Autodesk Fusion 360 part; units mm, degrees
(part 6 of 11)
extrude "Extrude4" cut sketch "Sketch2" against normal blind 3 contours L0 L603 L618 L619 L624 L628 L643 A50 L685 L691 L692 L696 L698 L700 L701 L702 L705 L707 L714 L715 L716 A52 L728 L732 L739 L740 L745 L748 L751 L756 L761 A55 L767 L768 L771 L774 L777 L784 L788 L797 L804 L808 L814 L817 L818 L825 L829 L831 A59 L832 L837 L838 L839 L844 L847 L854 L857 L858 L869 L873 L876 A60 L892 L900 L901 L905 L906 L907 L914 L918 L933 L937 L975 L977 L985 L986 L990 L1001 L1013 L1022 L1024 L1038 L1039 L1041 L1047 L1051 L1054 L1059 A65 L1077 L1080 L1082 L1085 L1091 L1098 L1101 L1102 L1115 A70 L1123 L1132 L1134 L1135 L1137 L1138 L1143 L1174 L1182 L1199 L1212 L1213 L1222 L1223 L1224 L1227 L1232 L1233 L1239 L1247 L1252 L1265 L1268 L1269 L1278 L1283 L1289 L1302 L1306 L1311 L1312 L1313 L1315 A78 L1324 L1327 L1329 A80 L1338 A81 L1341 L1344 L1347 L1348 A85 L1355 L1357 L1360 L1368 L1371 L1376 L1378 L1382 L1389 L1391 L1392 L1393 L1397 L1401 L1402 L1405 L1407 L1408 L1409 A89 L1418 L1419 L1420 L1422 L1426 L1427 L1430 L1431 L1433 L1436 L1438 L1441 L1442 L1444 L1445 L1446 L1447 L1460 L1470 L1471 L1478 L1484 L1485 L1486 L1498 L1499 L1501 L1502 L1507 L1511 L1541 L1548 L1552 L1556 L1572 L1574 L1575 L1582 L1585 L1586 L1587 L1588 L1596 A100 L1598 L1599 L1608 L1612 L1613 L1615 L1617 L1620 L1621 L1624 L1625 A102 L1632 L1634 L1635 L1637 L1638 L1641 L1642 L1644 L1645 L1647 L1650 L1652 L1655 L1659 L1660 L1662 L1664 L1666 L1669 L1671 L1672 L1673 L1674 L1676 L1677 L1678 L1681 L1682 L1687 L1688 A107 L1697 A108 L1699 L1700 L1710 L1711 L1713 L1714 L1715 L1716 L1718 L1719 L1722 L1723 L1726 L1728 L1729 L1730 L1731 L1735 L1736 A109 L1739 L1740 L1741 L1742 L1745 L1746 L1747 L1748 L1749 L1751 L1752 L1753 L1757 L1758 L1759 L1761 L1764 L1765 L1767 L1769 L1773 L1775 L1777 L1780 L1786 L1788 L1789 L1790 L1791 L1792 L1794 L1795 A114 L1797 A115 L1799 L1800 A116 A117 L1804 L1807 L1813 L1814 L1818 L1819 L1820 L1821 L1822 L1823 L1824 L1825 L1826 A119 L1827 L1828 L1829 L1830 L1831 L1832 L1833 A120 L1834 L1835 L1836 L1837 L1838 L1839 L1840 L1841 L1842 L1843 L1844 L1845 L1846 L1847 L1848 A121 L1849 L1850 L1851 L1852 L1853 L1854 L1855 L1856 A122 L1857 L1858 L1859 L1860 L1861 L1862 L1863 L1864 L1865 A123 L1866 L1867 L1868 L1869 L1870 L1871 L1872 L1873 L1874 L1875 L1876 A124 L1879 L1881 L1882 L1883 L1886 L1894 L1895 A126 L1904 L1905 L1906 L1910 L1918 L1919 L1921 L1922 L1923 L1925 L1932 L1934 L1935 L1936 L1937 L1938 L1939 A128 L1940 L1941 L1942 L1943 L1944 L1945 L1946 L1947 L1948 L1949 L1950 L1951 L1952 L1953 L1954 L1955 L1956 L1957 L1958 L1959 L1960 L1961 L1962 L1963 L1964 L1966 L1967 L1968 L1969 L1970 L1971 L1972 L1973 A129 L1974 L1975 L1976 L1977 L1978 L1979 L1980 L1981 L1982 L1983 L1984 L1985 L1986 L1987 A130 L1988 L1989 L1990 L1991 L1992 L1993 L1994 L1995 L1997 L1998 L2002 L2003 A131 L2004 L2006 L2007 L2009 L2011 L2012 L2013 L2014 L2016 L2017 L2021 L2023 L2024 L2025 L2026 L2027 L2028 L2030 L2031 L2032 L2033 L2034 L2035 L2036 L2037 L2038 L2039 L2040 L2041 L2042 L2045 A132 L2047 L2048 L2049 L2050 L2051 L2053 A133 L2055 L2056 L2057 L2060 L2062 L2063 L2064 L2066 L2067 L2069 L2071 L2072 L2073 L2074 L2075 L2076 L2077 L2078 L2080 L2081 L2082 L2084 L2085 L2086 L2088 L2089 L2091 L2092 L2095 L2096 L2097 L2098 L2099 L2100 L2103 L2104 L2105 L2106 L2107 L2111 L2113 L2114 L2115 L2116 L2117 L2118 L2119 L2120 L2121 L2122 L2123 L2124 L2125 L2126 L2129 L2130 L2131 L2133 L2134 L2135 L2136 A134 L2137 L2138 L2139 L2140 L2141 L2142 L2143 L2144 L2147 L2148 L2149 L2151 L2152 L2153 A135 L2155 L2156 L2157 A136 L2159 L2160 L2161 L2162 L2163 L2164 L2165 L2166 A137 L2167 L2169 L2171 L2172 L2173 L2174 L2175 L2176 L2178 L2179 L2180 L2181 L2182 L2184 L2185 L2186 L2188 L2189 L2190 L2191 L2192 L2193 L2194 L2195 L2196 L2197 L2198 A138 L2199 L2200 L2201 L2202 A140 A141 L2205 L2206 L2207 L2208 L2209 L2210 L2211 L2212 L2213 L2214 L2215 L2216 L2217 L2218 L2220 L2221 L2223 L2224 L2225 L2226 L2227 L2228 L2229 A142 L2230 L2233 L2234 L2235 L2236 L2237 L2238 A144 L2239 L2240 L2241 L2242 L2243 L2244 L2245 L2246 L2247 L2248 L2249 L2250 L2251 L2252 L2253 L2254 L2255 L2256 L2257 A145 L2258 L2259 L2260 L2261 L2262 L2263 L2264 L2265 L2266 L2267 L2268 L2269 L2270 L2271 L2272 L2273 L2274 L2275 A147 L2276 L2277 L2278 L2279 L2280 L2281 L2282 L2283 L2284 L2285 L2286 L2287 L2288 L2289 L2290 L2291 L2292 L2293 A149 L2294 L2295 L2296 A150 L2297 L2298 L2299 L2300 L2301 L2302 L2303 L2304 L2305 L2306 L2307 A151 L2308 L2309 L2310 L2311 L2312 L2313 L2314 L2315 L2316 L2317 L2318 L2319 L2320 L2321 L2322 L2323 L2324 L2325 L2326 L2327 L2328 L2329 L2330 L2331 L2332 L2333 L2334 L2335 L2336 L2337 L2338 L2883 L2884 L2885 L2886 L2887 L2888 L2889 L2890 L2891 A183 A200 L3160 L3161 L3162 L3163 L3164 L3165 L3166 L3167 L3168 | L0 L3 L619 L628 L643 L685 L1022 L1024 A65 L1077 L1080 L1082 L1085 L1091 L1098 L1101 L1102 L1115 A70 L1123 L1132 L1134 L1135 L1137 L1138 L1143 L1174 L1182 L1199 L1212 L1213 L1222 L1223 L1224 L1227 L1232 L1233 L1239 L1247 L1252 L1265 L1268 L1269 L1278 L1283 L1289 L1302 L1306 L1311 L1312 L1313 L1315 A78 L1324 L1327 L1329 L1338 A81 L1341 L1344 L1347 L1348 L1355 L1357 L1360 L1368 L1371 L1376 L1378 L1382 L1391 L1392 L1393 L1397 L1401 L1402 L1405 L1407 L1408 L1409 A89 L1418 L1420 L1422 L1427 L1430 L1433 L1438 L1441 L1444 L1445 L1446 L1447 L1460 L1470 L1471 L1478 L1484 L1485 L1486 L1498 L1499 L1501 L1502 L1507 L1728 L1731 L1736 L1746 L1747 L1749 L1751 L1758 L1764 L1777 L1789 L1794 L1795 L1799 A116 L1804 L1807 L1813 L1814 L1834 A124 L1882 A126 L1905 L1922 L1939 A128 L1941 L1942 L1944 L1947 L1948 L1949 L1950 L1951 L1952 L1954 L1955 L1956 L1957 L1966 L1967 L1971 L1973 L1974 L1977 L1978 L1980 L1981 L1983 L1984 L1985 L1986 A130 L1988 L1989 L1991 L1992 L1994 L1997 L2026 L2032 L2040 L2062 L2063 L2064 L2080 L2081 L2082 L2086 L2103 L2105 L2106 L2107 L2114 L2115 L2116 L2117 L2119 L2120 L2121 L2122 L2123 L2124 L2125 L2126 L2129 L2130 L2131 L2133 L2134 L2135 L2136 A134 L2137 L2138 L2139 L2140 L2141 L2142 L2143 L2144 L2147 L2148 L2149 L2151 L2152 L2153 A135 L2155 L2156 L2157 A136 L2159 L2160 L2161 L2162 L2163 L2164 L2165 L2166 A137 L2167 L2169 L2171 L2172 L2173 L2174 L2175 L2176 L2178 L2179 L2180 L2181 L2182 L2184 L2185 L2186 L2193 L2194 L2195 L2196 L2197 L2198 A138 L2199 L2200 L2201 L2202 L2205 L2207 L2208 L2209 L2210 L2211 L2212 L2214 L2215 L2216 L2217 L2218 L2220 L2224 L2225 L2230 L2233 L2234 L2235 L2236 L2237 L2238 A144 L2254 L2255 L2256 L2257 A145 L2258 L2262 L2263 L2267 L2268 L2269 L2270 L2271 L2273 L2274 L2275 L2276 L2278 L2279 L2280 L2281 L2282 L2283 L2284 L2285 L2291 L2292 L2293 A149 L2294 L2295 A150 L2297 L2298 L2299 L2300 L2301 L2302 A151 L2308 L2309 L2320 L2321 L2324 L2331 L2332 L2333 L2436 L2437 L2438 A158 A173 L2690 L2691 L2692 L2693 L2694 A174 L2695 L2696 L2697 L2698 L2699 L2700 L2701 L2702 L2703 L2704 A175 L2705 L2706 L2707 L2708 L2709 L2727 L2728 L2729 L2730 L2731 A176 L2732 L2733 L2734 L2735 L2736 L2737 L2738 L2739 L2740 L2741 A177 L2742 L2743 L2744 L2745 L2746 L2764 L2765 L2766 L2767 L2768 A178 L2769 L2770 L2771 L2772 L2773 L2774 L2775 L2776 L2777 L2778 A179 L2779 L2780 L2781 L2782 L2783 L2801 L2802 L2803 L2804 L2805 A180 L2806 L2807 L2808 L2809 L2810 L2811 L2812 L2813 L2814 L2815 A181 L2816 L2817 A200 | L0 L1820 L1821 L1822 L1823 L1824 A119 L1829 L1830 L1833 A120 L1836 L1837 L1838 L1839 L1842 L1843 L1844 L1845 L1848 L1849 L1850 L1852 L1855 L1858 L1859 L1860 L1861 L1862 L1865 A123 L1866 L1867 L1868 L1869 L1873 L1876 L2260 L2261 L2264 L2265 L2266 L2272 A147 L2277 L2286 L2287 L2288 L2289 L2296 L2303 L2304 L2306 L2307 L2310 L2312 L2313 L2314 L2315 L2316 L2317 L2318 L2322 L2323 L2325 L2328 L2329 L2330 L2334 L2335 L2336 L2337 L2338 L2462 L2463 A159 L2464 L2465 L2466 L2467 L2468 L2469 L2470 L2471 L2472 L2473 A160 L2474 L2475 | L0 L603 L618 L624 A50 L691 L692 L696 L698 L700 L701 L702 L705 L707 L714 L715 L716 A52 L728 L732 L739 L740 L745 L748 L751 L756 L761 A55 L767 L768 L771 L774 L777 L784 L788 L797 L804 L808 L814 L817 L818 L825 L829 L831 A59 L832 L837 L838 L839 L844 L847 L854 L857 L858 L869 L873 L876 A60 L892 L900 L901 L905 L906 L907 L914 L918 L933 L937 L975 L977 L985 L986 L990 L1001 L1013 L1038 L1039 L1041 L1047 L1051 L1054 L1059 A80 A85 L1511 L1541 L1572 L1574 L1575 L1582 L1585 L1586 L1587 L1588 A100 L1598 L1608 L1612 L1613 L1615 L1620 L1621 L1624 L1625 A102 L1632 L1634 L1635 L1637 L1638 L1641 L1642 L1644 L1645 L1647 L1650 L1652 L1655 L1659 L1660 L1662 L1664 L1666 L1669 L1671 L1672 L1673 L1674 L1676 L1677 L1678 L1681 L1682 L1687 L1688 A107 L1697 A108 L1699 L1700 L1710 L1711 L1713 L1714 L1715 L1716 L1718 L1719 L1722 L1723 L1726 L1729 L1735 L1739 L1740 L1741 L1742 L1745 L1752 L1753 L1759 L1786 L1792 L1800 L1818 L1819 L1825 L1827 L1828 L1835 L1840 L1846 L1847 A121 L1851 L1853 L1854 L1856 A122 L1857 L1863 L1864 L1870 L1871 L1874 L1879 L1881 L1883 L1886 L1894 L1895 L1904 L1906 L1910 L1918 L1919 L1921 L1923 L1925 L1932 L1934 L1936 L1937 L1938 L1940 L1943 L1945 L1946 L1953 L1958 L1959 L1960 L1962 L1963 L1964 L1968 L1969 L1970 L1972 A129 L1975 L1976 L1979 L1982 L1987 L1990 L1993 L1995 L1998 L2002 A131 L2004 L2006 L2007 L2009 L2011 L2012 L2013 L2014 L2016 L2017 L2021 L2023 L2025 L2028 L2030 L2031 L2033 L2034 L2036 L2037 L2038 L2039 L2041 L2045 A132 L2047 L2048 L2051 A133 L2055 L2056 L2057 L2060 L2066 L2067 L2069 L2071 L2072 L2073 L2074 L2075 L2076 L2077 L2078 L2084 L2085 L2088 L2089 L2091 L2092 L2095 L2096 L2097 L2098 L2099 L2100 L2104 L2111 L2113 L2118 L2188 L2189 L2190 L2191 L2192 A140 A141 L2206 L2213 L2221 L2223 L2226 L2227 L2228 L2229 A142 L2239 L2240 L2241 L2242 L2243 L2244 L2245 L2246 L2247 L2248 L2249 L2250 L2251 L2252 L2253 L2290 A161 L2489 L2490 L2491 L2492 L2493 L2494 L2495 L2496 L2497 L2498 L2499 L2500 L2501 L2502 L2503 A162 L2504 L2505 L2506 L2507 L2508 L2509 L2510 L2511 L2512 L2513 A163 L2514 L2515 L2516 L2517 L2518 L2519 L2520 L2521 L2522 L2523 L2524 L2525 L2526 L2527 L2528 L2529 L2530 L2531 L2532 L2533 L2534 L2535 L2536 L2537 L2538 L2539 L2540 A164 L2541 L2542 L2543 L2544 L2545 L2546 L2547 L2548 L2549 L2550 A165 L2551 L2552 L2553 L2554 L2555 L2556 L2557 L2558 L2559 L2560 L2561 L2562 L2563 L2564 L2565 L2566 L2567 L2568 L2569 L2570 L2571 L2572 L2573 L2574 L2575 L2576 L2577 A166 L2578 L2579 L2580 L2581 L2582 L2583 L2584 L2585 L2586 L2587 A167 L2588 L2589 L2590 L2591 L2592 L2593 L2594 L2595 L2596 L2597 L2598 L2599 L2600 L2601 L2602 L2603 L2604 L2605 L2606 L2607 L2608 L2609 L2610 L2611 L2612 L2613 L2614 A168 L2615 L2616 L2617 L2618 L2619 L2620 L2621 L2622 L2623 L2624 A169 L2625 L2626 L2627 L2628 L2629 L2630 L2631 L2632 L2633 L2634 L2635 L2636 L2637 L2638 L2639 A170 A183 | L3 A2 A3 L223 L238 L240 A19 L245 A20 L246 L337 L338 L341 L343 L344 L345 L346 L347 L348 L350 L352 L385 L386 L387 L388 L389 L390 L391 L392 L393 L394 L395 L396 L397 L398 L399 L400 L403 L405 L407 L413 L414 L415 L416 A32 L417 L418 L419 L420 L421 A33 L422 L423 L424 L425 L428 L429 L430 L432 L433 L434 L435 L441 L442 L443 A34 L445 L446 L447 L450 L451 L452 L453 L454 L455 L456 L457 L459 L460 L462 L463 L464 L466 A35 L467 L468 L469 L470 L471 L472 L473 L474 L475 L476 L477 L478 L479 L480 L481 L482 L497 L498 L499 L500 L501 L502 L503 L504 L505 L506 L507 L508 L509 L510 L511 L512 L513 L514 L515 L516 L625 L638 L639 L763 L764 L769 L775 A56 L798 L811 L815 L816 L820 L821 A58 L824 L826 L828 L830 L833 L835 L845 L849 L852 L859 L861 L862 L863 L866 L867 L870 L875 L883 L891 L893 L898 L908 L911 L915 L919 L921 L929 L934 L1020 L1034 L1044 L1050 L1052 L1058 L1066 L1078 L1079 L1083 L1086 L1087 L1088 L1089 L1092 A67 L1093 L1094 L1095 L1096 L1099 L1103 L1107 L1108 L1110 L1111 L1112 L1113 L1114 L1118 A69 L1122 L1124 L1125 L1126 L1127 L1128 L1129 L1130 L1131 L1136 L1144 L1145 L1147 L1148 L1151 L1152 A71 L1155 L1157 A72 L1168 L1170 L1173 L1177 L1178 L1179 L1181 L1187 L1188 L1195 L1200 L1204 L1206 L1207 L1211 L1214 L1216 L1218 L1221 L1225 L1230 L1236 L1246 L1248 L1253 L1275 L1296 L1888 A125 A127 L1924 A173 A193 L3056 L3057 L3058 L3059 L3060 A194 L3061 L3062 L3063 L3064 L3065 L3066 L3067 L3068 L3069 L3070 A195 L3071 L3072 L3073 L3074 L3075 L3093 L3094 L3095 L3096 L3097 A196 L3098 L3099 L3100 L3101 L3102 L3103 L3104 L3105 L3106 L3107 A197 L3108 L3109 L3110 L3111 L3112 L3130 L3131 L3132 L3133 L3134 A198 L3135 L3136 L3137 L3138 L3139 L3140 L3141 L3142 L3143 L3144 A199 L3145 L3146 L3147 L3148 L3149 A200 A222 | A124 A125 A126 A127 A173 A200 | L2 L77 L80 L81 L84 L85 L89 L123 L124 L125 L126 L127 L128 L129 L130 L131 L132 L133 L134 L135 L136 L137 L138 L139 L140 L141 L142 L143 L144 L145 L146 L147 L148 L149 L150 A8 A10 L185 L187 A12 L188 A13 L190 L191 L192 L193 L194 L195 L196 A14 L197 L198 L199 L200 L201 L202 L203 L204 L205 L206 L207 L208 L209 L210 A15 L211 L212 L213 L214 L215 L216 L217 L218 L219 L220 L221 L224 L225 L226 L227 L228 L229 L230 L231 L232 L233 L234 L235 L236 L249 L250 L251 L252 L253 L254 L255 L256 L257 L258 L259 L260 A36 L544 A39 L545 L571 L572 L620 L621 L631 L633 L637 A46 A47 L641 L656 L663 L671 L674 L693 L695 L703 L706 L709 L711 L713 L724 L726 L727 L730 L733 L738 L741 L746 A53 L749 L750 A54 L754 L755 L757 L758 L759 L760 L762 L766 L770 L772 L773 L776 L778 L779 L780 L781 L782 L786 L787 L789 L791 L792 L793 L794 L795 L796 L799 L800 L801 L802 L803 A57 L805 L806 L807 L809 L810 L812 L813 L819 L822 L823 L827 L834 L836 L840 L841 L843 L846 L848 L850 L851 L853 L855 L860 L864 L865 L868 L871 L872 L874 L877 L879 L899 L902 L909 L913 L917 L920 L930 L931 L944 L945 L1081 L1084 A66 A68 L1097 L1105 L1109 L1116 L1119 L1120 L1121 L1133 L1139 L1140 L1141 L1142 L1146 L1153 L1156 L1160 L1161 L1162 L1163 L1164 L1166 L1167 L1169 L1172 L1176 L1183 L1184 L1185 L1186 L1189 L1190 L1191 L1192 L1193 L1196 L1197 A73 L1201 L1203 L1208 L1209 L1210 L1215 L1217 L1219 L1220 L1226 L1228 L1229 L1234 L1237 L1240 L1241 L1242 L1243 L1244 L1245 L1249 L1251 L1255 L1273 A77 A90 L1440 L1483 L1503 L2376 L2377 L2378 L2379 L2380 L2381 L2384 L2385 L2386 L2387 L2388 A154 L2389 L2390 L2391 L2392 L2393 L2394 L2395 L2396 L2397 L2398 L2399 L2400 L2401 L2403 L2404 L2406 A155 L2407 L2408 L2409 L2410 L2411 L2412 L2413 L2414 L2415 L2417 L2418 L2420 L2421 A190 L3216 L3217 L3218 L3219 L3220 L3221 L3222 L3223 L3224 L3225 L3226 L3227 A202 L3228 L3229 L3230 L3231 L3232 L3233 L3234 L3235 L3236 L3237 A203 L3238 L3239 L3240 L3241 L3242 L3243 L3244 L3245 L3246 L3247 L3248 L3249 L3250 L3251 L3252 L3253 L3254 L3255 L3256 L3257 L3258 L3259 L3260 L3261 L3262 L3263 L3264 A204 L3265 L3266 L3267 L3268 L3269 L3270 L3271 L3272 L3273 L3274 A205 L3275 L3276 L3277 L3278 L3279 L3280 L3281 L3282 L3283 L3284 L3285 L3286 L3287 L3288 L3289 L3290 L3291 L3292 L3293 L3294 L3295 L3296 L3297 L3298 L3299 L3300 L3301 A206 L3302 L3303 L3304 L3305 L3306 L3307 L3308 L3309 L3310 L3311 A207 L3312 L3313 L3314 L3315 L3316 L3317 L3318 L3319 L3320 L3321 L3322 L3323 L3324 L3325 L3326 L3327 L3328 L3329 L3330 L3331 L3332 L3333 L3334 L3335 L3336 L3337 L3338 A208 L3339 L3340 L3341 L3342 L3343 L3344 L3345 L3346 L3347 L3348 A209 L3349 L3350 L3351 L3352 L3353 L3354 L3355 L3356 L3357 L3358 L3359 L3360 L3361 L3362 L3363 A210 A225 L3595 L3596 L3597 | L1387 L1390 L1412 L1423 L1424 L1435 L1437 L1443 L1877 L1880 L1884 L1887 L1891 L1892 A125 L1893 L1896 L1901 L1903 L1911 L1912 L1913 A127 L1916 L1917 L1926 L1929 L1930 L1931 L1933 L2671 L2672 L2673 L2674 L2675 L2676 L2677 L2678 L2679 A173 | A2 A3 L29 L30 L34 L37 L40 L43 L98 L107 L116 L117 L122 L171 A9 A11 L222 L223 L237 L238 L239 L240 L241 L242 L243 A18 A19 L244 L245 A20 L246 A21 L247 L248 L261 L262 L266 L268 L270 L271 L272 L273 L274 L275 L276 L277 L278 L279 L280 L281 L282 L283 L284 L285 L286 L287 L288 L289 L290 L291 L292 L294 A22 L295 L296 A23 L297 L298 L299 L300 L301 L302 L303 L304 L305 L306 L307 L308 L309 L310 L311 L312 L313 L314 L315 L316 A24 L317 L318 A25 L319 L320 L321 L322 L323 A26 L324 L325 L326 L327 L328 L329 L330 A27 L331 L332 L333 L334 L335 L336 L337 L338 L339 A28 L340 L341 L342 L343 L344 L345 L346 L347 L348 L349 L350 L351 L352 L353 L354 L355 L356 L357 L358 L359 L360 L361 L362 L363 L364 L365 L366 L367 L368 L369 L370 L371 L372 L373 L374 L375 L376 L377 L379 L380 L382 L383 L384 L385 L386 L387 L388 L389 L390 L391 L392 L393 L394 L395 L396 L397 L398 L399 L400 L401 L402 L403 L404 L405 L406 L407 L408 L409 L410 L411 L412 A31 L413 L414 L415 L416 A32 L417 L418 L419 L420 L421 A33 L422 L423 L424 L425 L428 L429 L430 L432 L433 L434 L435 L441 L442 L443 A34 L445 L446 L447 L450 L451 L452 L453 L454 L455 L456 L457 L459 L460 L462 L463 L464 L466 A35 L467 L468 L469 L470 L471 L472 L473 L474 L475 L476 L477 L478 L479 L480 L481 L482 L497 L498 L499 L500 L501 L502 L503 L504 L505 L506 L507 L508 L509 L510 L511 L512 L513 L514 L515 L516 L546 L547 L548 L549 L550 L551 L552 L553 L554 L555 L556 L557 L558 L559 L562 L563 L565 A41 L566 A42 L573 L578 L581 L582 L585 L586 L587 L589 L590 L591 L592 L594 L596 L597 L598 L600 L601 L604 L605 L606 L608 L609 L610 L611 L612 L615 L625 L638 L639 L644 L645 L647 L648 L649 L650 L651 A48 L652 L654 L655 L658 L659 L665 L666 L667 L668 L669 L670 L672 L673 L675 L676 L677 L678 L679 L681 L682 L683 L684 L686 A51 L687 L688 L690 L718 L720 L721 L725 L729 L735 L737 L747 L753 L763 L764 L765 L769 L775 L790 A56 L798 L811 L815 L816 L820 L821 A58 L824 L826 L828 L830 L833 L835 L845 L849 L852 L859 L861 L862 L863 L866 L867 L870 L875 L881 L883 L884 L891 L893 L898 L908 L911 L915 L919 L921 L929 L934 L939 L940 L941 L942 L943 L946 L950 L951 L953 A62 L956 L960 L961 L962 L964 L965 L968 L969 L970 L976 L978 L981 L987 A63 L988 L991 L992 L993 L997 L1000 L1002 L1003 L1006 L1007 L1009 L1011 L1012 L1014 L1020 L1034 L1036 L1044 L1050 L1052 L1056 L1058 L1060 L1066 L1068 L1078 L1079 L1083 L1086 L1087 L1088 L1089 L1092 A67 L1093 L1094 L1095 L1096 L1099 L1103 L1107 L1108 L1110 L1111 L1112 L1113 L1114 L1118 A69 L1122 L1124 L1125 L1126 L1127 L1128 L1129 L1130 L1131 L1136 L1144 L1145 L1147 L1148 L1149 L1150 L1151 L1152 A71 L1154 L1155 L1157 L1158 A72 L1159 L1165 L1168 L1170 L1171 L1173 L1175 L1177 L1178 L1179 L1181 L1187 L1188 L1195 L1200 L1204 L1206 L1207 L1211 L1214 L1216 L1218 L1221 L1225 L1230 L1236 L1246 L1248 L1253 L1254 L1261 L1275 L1276 L1296 L1314 L1322 A79 A82 L1340 L1346 A84 A86 L1374 L1403 L1411 L1416 L1434 L1435 L1443 L1527 L1546 L1551 L1570 L1584 L1589 L1602 L1623 A110 A118 L1888 A125 A127 L1924 L2010 L2015 L2029 L2046 L2359 A170 L2640 L2641 L2642 L2643 L2644 L2645 L2646 L2647 L2648 L2671 L2672 L2673 L2674 L2675 L2676 L2677 L2678 L2679 A173 A222 L3555 L3556 L3557 L3558 L3559 L3560 L3561 L3562 L3563 L3586 L3587 L3588 L3589 L3590 L3591 L3592 L3593 L3594 A225 | L1388 L1389 L1398 L1417 L1421 L1428 L1429 L1442 A124 L1889 L1890 L1892 L1896 L1897 L1898 A126 L1899 L1900 L1902 L1903 L1907 L1911 L1915 L1917 L1920 L1927 L1928 L1929 L1931 L1933 A200 L3160 L3161 L3162 L3163 L3164 L3165 L3166 L3167 L3168 | L2 L4 L5 L6 L7 L8 L9 L10 L11 L12 L13 L14 L15 A0 A1 L22 L32 L36 L38 L42 L44 L49 L52 L54 L75 L76 L77 A4 A5 L78 L79 L80 L81 L82 L83 L84 L85 A6 L86 L87 L88 L89 L90 A7 L91 L92 L106 L112 L114 L120 L121 L123 L124 L125 L126 L127 L128 L129 L130 L131 L132 L133 L134 L135 L136 L137 L138 L139 L140 L141 L142 L143 L144 L145 L146 L147 L148 L149 L150 L151 L152 L153 L154 L155 L156 L172 A8 A10 L185 L187 A12 L188 A13 L190 L191 L192 L193 L194 L195 L196 A14 L197 L198 L199 L200 L201 L202 L203 L204 L205 L206 L207 L208 L209 L210 A15 L211 L212 L213 L214 L215 L216 L217 L218 L219 L220 L221 L224 L225 L226 L227 L228 L229 L230 L231 L232 L233 L234 L235 L236 L249 L250 L251 L252 L253 L254 L255 L256 L257 L258 L259 L260 L517 L518 L519 L520 L521 L522 L523 L525 L526 L527 L528 L530 L531 L532 L535 L537 L538 L539 A36 L541 L542 L543 A37 L544 A38 A39 L545 L560 A40 L561 L564 L567 L568 L569 L571 L572 L574 L575 L576 L577 L579 L580 L583 L584 A43 L588 L593 L595 L599 L602 L607 L613 L614 L616 L620 L621 L629 L631 L632 L633 L635 L636 L637 A46 A47 L641 L646 L656 L662 L663 L671 L674 A49 L689 L693 L695 L703 L706 L709 L711 L713 L724 L726 L727 L730 L733 L738 L741 L746 A53 L749 L750 A54 L754 L755 L757 L758 L759 L760 L762 L766 L770 L772 L773 L776 L778 L779 L780 L781 L782 L786 L787 L789 L791 L792 L793 L794 L795 L796 L799 L800 L801 L802 L803 A57 L805 L806 L807 L809 L810 L812 L813 L819 L822 L823 L827 L834 L836 L840 L841 L843 L846 L848 L850 L851 L853 L855 L860 L864 L865 L868 L871 L872 L874 L877 L879 L899 L902 L909 L913 L917 L920 L930 L931 L944 L945 L955 L958 L959 L963 L966 L967 L971 L973 L974 L979 L983 L1004 L1005 L1016 L1017 L1018 L1019 L1028 L1029 L1030 L1032 L1035 L1037 L1045 L1046 L1048 L1049 L1055 L1057 L1062 L1063 L1064 L1065 L1067 L1069 L1071 L1074 L1075 L1076 L1081 L1084 A66 A68 L1097 L1105 L1109 L1116 L1119 L1120 L1121 L1133 L1139 L1140 L1141 L1142 L1146 L1153 L1156 L1160 L1161 L1162 L1163 L1164 L1166 L1167 L1169 L1172 L1176 L1183 L1184 L1185 L1186 L1189 L1190 L1191 L1192 L1193 L1196 L1197 A73 L1198 L1201 L1203 L1208 L1209 L1210 L1215 L1217 L1219 L1220 L1226 L1228 L1229 L1231 L1234 L1235 L1237 L1240 L1241 L1242 L1243 L1244 L1245 L1249 L1251 L1255 L1257 L1264 L1266 L1270 L1271 L1273 L1277 L1280 L1282 L1285 A77 L1291 L1294 L1295 L1297 L1298 L1299 L1300 L1301 L1303 L1304 L1305 L1308 L1309 L1317 L1319 L1323 L1325 L1326 L1328 L1331 L1332 L1333 L1334 L1336 L1337 L1339 L1342 L1343 L1345 L1349 A83 L1350 L1351 L1353 L1359 L1361 L1362 L1363 L1364 L1365 L1366 A88 L1370 L1372 L1373 L1375 L1377 L1379 L1380 L1381 L1383 L1384 L1385 L1386 L1396 L1400 L1404 L1410 L1413 L1414 L1415 L1425 A90 L1439 A91 L1440 L1449 L1450 A92 L1452 L1453 L1455 L1456 L1457 L1461 L1464 L1465 L1466 L1468 L1469 L1473 L1474 L1475 A93 L1479 L1480 L1481 L1482 L1483 L1487 L1488 L1491 L1492 L1493 L1496 A94 L1500 L1503 L1505 L1508 L1509 L1513 L1514 L1515 L1517 A96 L1518 L1519 L1520 L1522 L1523 L1524 A97 A98 L1528 L1531 L1533 L1534 L1536 L1537 L1540 L1545 L1547 L1549 L1550 L1553 L1554 L1555 L1557 L1562 L1563 L1564 L1565 L1567 L1569 L1571 L1573 L1578 L1581 L1583 L1590 L1591 L1592 L1597 L1600 L1603 L1604 L1606 L1607 L1609 L1610 A101 L1618 L1622 L1626 L1627 L1628 L1629 L1630 L1631 L1633 L1636 L1639 L1640 L1643 L1646 A103 L1648 L1649 L1651 L1653 L1654 L1656 L1657 L1658 L1661 L1663 L1665 L1667 L1668 A104 A105 L1670 L1675 L1679 L1680 L1683 L1684 L1685 L1686 L1689 L1690 L1695 L1696 L1698 L1701 L1703 L1705 L1706 L1709 L1717 L1720 L1721 L1724 L1725 L1733 L1734 L1737 L1738 L1743 L1750 L1754 L1755 L1756 L1760 L1762 L1763 A111 L1766 L1768 L1770 L1771 L1772 L1776 L1778 A112 L1779 L1782 L1783 L1784 L1787 L1796 L1798 L1801 L1802 L1803 L1805 L1808 L1809 L1810 L1811 L1812 L1815 L1817 L2339 L2340 L2341 L2342 L2343 A152 L2344 L2345 L2346 L2347 L2348 A153 L2349 L2350 L2351 L2352 L2353 L2354 L2355 L2356 L2357 L2358 L2360 L2361 L2362 L2363 L2364 L2365 L2366 L2367 L2368 L2369 L2370 L2371 L2372 L2373 L2374 L2375 L2376 L2377 L2378 L2379 L2380 L2381 L2382 L2383 L2384 L2385 L2386 L2387 L2388 A154 L2389 L2390 L2391 L2392 L2393 L2394 L2395 L2396 L2397 L2398 L2399 L2400 L2401 L2403 L2404 L2406 A155 L2407 L2408 L2409 L2410 L2411 L2412 L2413 L2414 L2415 L2417 L2418 L2420 L2421 L2422 L2423 L2426 L2429 L2431 L2433 L2434 L2435 A190 L3006 L3007 L3008 L3009 L3010 L3011 L3012 L3013 L3014 L3037 L3038 L3039 L3040 L3041 L3042 L3043 L3044 L3045 A193 | L1387 L1388 L1389 L1390 L1398 L1412 L1417 L1421 L1423 L1424 L1428 L1429 L1435 L1437 L1442 L1443 L1877 L1880 L1884 L1887 L1889 L1890 L1891 L1893 L1897 L1898 L1899 L1900 L1901 L1902 L1907 L1912 L1913 L1915 L1916 L1920 L1926 L1927 L1928 L1930 L2667 L2668 L2669 L2670 L3169 L3170 L3171 L3172 | L2 L1257 L1266 L1270 L1280 L1297 L1298 L1299 L1300 L1305 L1308 L1309 L1317 L1323 L1328 L1332 L1334 L1337 L1343 A83 L1350 L1361 L1363 A88 L1370 L1372 L1373 L1379 L1381 L1384 L1404 L1410 L1439 L1479 L1491 L1492 L1515 L1518 L1520 L1528 L1531 L1540 L1590 L1591 L1607 L1609 L1610 A101 L1622 L1627 L1628 L1630 L1631 L1639 L1640 L1646 L1649 L1653 L1656 L1657 L1663 L1665 L1668 A105 L1679 L1684 L1686 L1701 L1720 L1734 L1738 L1743 L1815 L3377 L3378 A211 L3379 L3380 L3381 L3382 L3383 L3384 L3385 L3386 L3387 L3388 A212 L3389 L3390 | L3 A193 A222 | L2 L3 L4 L5 L6 L7 L8 L9 L10 L11 L12 L13 L14 L15 A0 A1 L22 L151 L152 L155 L156 L517 L518 L519 L520 L521 L522 L523 L525 L526 L527 L528 L530 L531 L532 L535 L537 L538 L539 L541 L542 L543 A37 A38 L560 A40 L561 L564 L567 L568 L569 L574 L575 L576 L577 L579 L580 L583 L584 A43 L588 L593 L595 L599 L602 L607 L613 L614 L616 L629 L632 L635 L636 L646 L662 A49 L689 L955 L958 L959 L963 L966 L967 L971 L973 L974 L979 L983 L1004 L1005 L1016 L1017 L1018 L1019 L1028 L1029 L1030 L1032 L1035 L1037 L1045 L1046 L1048 L1049 L1055 L1057 L1062 L1063 L1064 L1065 L1067 L1069 L1071 L1074 L1075 L1076 L1264 L1271 L1277 L1282 L1285 L1291 L1294 L1295 L1301 L1304 L1319 L1325 L1326 L1331 L1333 L1336 L1339 L1342 L1345 L1349 L1351 L1353 L1359 L1362 L1364 L1365 L1366 L1375 L1377 L1380 L1383 L1385 L1386 L1396 L1400 L1413 L1414 L1415 L1425 A91 L1449 L1450 A92 L1452 L1453 L1455 L1456 L1461 L1464 L1465 L1466 L1468 L1469 L1473 L1474 L1475 A93 L1480 L1481 L1482 L1487 L1493 L1496 A94 L1500 L1505 L1508 L1509 L1513 L1514 L1517 A96 L1519 L1522 L1523 L1524 A97 A98 L1533 L1534 L1536 L1537 L1545 L1547 L1549 L1550 L1553 L1554 L1555 L1557 L1562 L1563 L1564 L1565 L1567 L1569 L1571 L1573 L1578 L1581 L1583 L1592 L1597 L1600 L1603 L1604 L1618 L1626 L1629 L1633 L1643 A103 L1648 L1651 L1654 L1658 L1661 L1667 A104 L1670 L1675 L1680 L1683 L1685 L1689 L1690 L1695 L1696 L1698 L1703 L1705 L1706 L1717 L1721 L1724 L1725 L1733 L1737 L1750 L1754 L1755 L1756 L1760 L1762 L1763 A111 L1766 L1768 L1770 L1771 L1772 L1776 A112 L1779 L1782 L1783 L1784 L1787 L1796 L1798 L1801 L1802 L1803 L1805 L1808 L1810 L1811 L1812 L2339 L2340 L2341 L2342 L2343 A152 L2344 L2345 L2346 L2347 L2348 A153 L2349 L2350 L2351 L2352 L2353 L2354 L2357 L2358 L2361 L2363 L2364 L2366 L2367 L2368 L2370 L2371 L2372 L2373 L2374 L2375 L2422 L2423 L2426 L2429 L2431 L2433 L2434 L2435 A193 A213 L3414 L3415 L3416 L3417 L3418 A214 L3419 L3420 L3421 L3422 L3423 L3424 L3425 L3426 L3427 L3428 A215 L3429 L3430 L3431 L3432 L3433 L3451 L3452 L3453 L3454 L3455 A216 L3456 L3457 L3458 L3459 L3460 L3461 L3462 L3463 L3464 L3465 A217 L3466 L3467 L3468 L3469 L3470 L3488 L3489 L3490 L3491 L3492 A218 L3493 L3494 L3495 L3496 L3497 L3498 L3499 L3500 L3501 L3502 A219 L3503 L3504 L3505 L3506 L3507 L3525 L3526 L3527 L3528 L3529 A220 L3530 L3531 L3532 L3533 L3534 L3535 L3536 L3537 L3538 L3539 A221 L3540 L3541 L3542 L3543 L3544 A222 | A0 A1 A2 A3 A193 A222 | A0 A1 L16 L17 L20 L21 L23 L24 L25 L26 L27 L28 L31 L32 L33 L39 L46 L47 L53 L54 L55 L58 L60 L61 L64 L65 L67 L69 L71 L73 L3037 L3038 L3039 L3040 L3041 L3042 L3043 L3044 L3045 A193 | L16 L18 L19 A2 L21 L23 L24 A3 L25 L26 L27 L28 L29 L35 L40 L41 L45 L48 L50 L51 L56 L57 L59 L62 L63 L66 L68 L70 L72 L74 A222 L3555 L3556 L3557 L3558 L3559 L3560 L3561 L3562 L3563 | L651 L652 L672 L683 L956 L962 L1149 L1150 L1154 L1158 L1159 L1165 L1171 L1175 L1254 L1261 A79 A82 L1340 L1374 L1403 L1411 L1416 L1434 L1435 L1443 L1527 L1546 L1551 L1570 L1584 L1589 L1602 L1623 A110 A118 L2010 L2015 L2029 L2046 L2649 L2650 L2651 L2652 L2667 L2668 L2669 L2670 L2872 L2873 L2874 L2875 L2876 A182 L2877 L2878 L3173 L3174 A201 L3175 L3176 L3177 L3178 L3179 | L1389 L1419 L1426 L1431 L1436 L1442 L1548 L1552 L1556 L1596 L1599 L1617 L1730 A109 L1748 L1757 L1761 L1765 L1767 L1769 L1773 L1775 L1780 L1788 L1790 L1791 A114 L1797 A115 A117 L1935 L1961 L2003 L2024 L2027 L2035 L2042 L2049 L2050 L2053 L2653 L2654 A171 L2655 L2656 L2657 L2658 L2659 L2660 L2661 L2662 L2663 L2664 A172 L2665 L2666 L2879 L2880 L2881 L2882 L3169 L3170 L3171 L3172 | L17 L18 L19 L20 L29 L31 L32 L33 L35 L39 L40 L41 L45 L46 L47 L48 L50 L51 L53 L54 L55 L56 L57 L58 L59 L60 L61 L62 L63 L64 L65 L66 L67 L68 L69 L70 L71 L72 L73 L74 L3033 L3034 L3035 L3036 L3564 L3565 L3566 L3567 | L32 L36 L38 L42 L44 L49 L52 L54 L75 L76 A4 A5 L78 L79 L82 L83 A6 L86 L87 L88 L90 A7 L91 L92 L106 L112 L114 L120 L121 L153 L154 L172 L2355 L2356 L2360 L2362 L2365 L2369 L2382 L2383 L3015 L3016 L3017 L3018 L3033 L3034 L3035 L3036 L3568 L3569 A223 L3570 L3571 L3572 L3573 L3574 L3575 L3576 L3577 L3578 L3579 A224 L3580 L3581 | L29 L30 L34 L37 L40 L43 L98 L107 L116 L117 L122 L171 L239 L242 L243 L244 L315 A24 L317 A25 L321 L322 L324 L331 L339 A28 L340 L342 L349 L351 L401 L402 L404 L406 L408 L409 L410 L411 L412 A31 L3019 L3020 A191 L3021 L3022 L3023 L3024 L3025 L3026 L3027 L3028 L3029 L3030 A192 L3031 L3032 L3564 L3565 L3566 L3567 L3582 L3583 L3584 L3585 | L1307 L1320 L1321 L1330 L1335 A84 L1352 L1354 A86 L1369 L1451 L1454 L1459 L1463 L1489 L1494 L1521 L1526 L1532 L1535 L1539 L1542 L1546 L1568 L1589 L1594 L1601 L1605 L1611 L1619 A170 L2640 L2641 L2642 L2643 L2644 L2645 L2646 L2647 L2648 | L1451 L1454 L1458 L1459 L1463 L1467 L1489 L1490 L1494 L1495 L1497 L1504 L1506 L1521 L1526 L1529 L1530 L1532 L1535 L1539 L1542 L1544 L1546 L1548 L1556 L1568 L1576 L1577 L1579 L1580 L1589 L1593 L1594 L1595 L1601 L1605 L1611 L1614 L1616 L1619 L2649 L2650 L2651 L2652 L2879 L2880 L2881 L2882 | L1307 L1320 L1321 L1330 L1335 A80 L1352 L1354 A85 L1369 L1458 L1467 L1490 L1495 L1497 L1504 L1506 L1529 L1530 L1544 L1548 L1556 L1576 L1577 L1579 L1580 L1593 L1595 L1614 L1616 L2883 L2884 L2885 L2886 L2887 L2888 L2889 L2890 L2891 A183 | L93 L97 L99 L101 L103 L105 L106 L111 L114 L115 L118 L119 L159 L162 L163 L166 L167 L168 L170 L173 A8 A10 L174 L175 L176 L177 L178 L179 L180 L181 A190 L3006 L3007 L3008 L3009 L3010 L3011 L3012 L3013 L3014 | L93 L94 L95 L96 L97 L99 L100 L101 L102 L103 L104 L105 L106 L107 L108 L109 L110 L111 L113 L114 L115 L116 L118 L119 L157 L158 L159 L160 L161 L162 L163 L164 L165 L166 L167 L168 L169 L170 L173 L182 L3015 L3016 L3017 L3018 L3582 L3583 L3584 L3585 | L94 L95 L96 L100 L102 L104 L107 L108 L109 L110 L113 L116 L157 L158 L160 L161 L164 L165 L169 A9 L174 L175 L176 L177 A11 L178 L179 L180 L181 L182 L3586 L3587 L3588 L3589 L3590 L3591 L3592 L3593 L3594 A225 | A80 A84 A85 A86 A170 A183 | A9 A11 L222 L237 L241 A18 A21 L247 L248 L261 L262 L266 L268 L270 L271 L272 L273 L274 L275 L276 L277 L278 L279 L280 L281 L282 L283 L284 L285 L286 L287 L288 L289 L290 L291 L292 L294 A22 L295 L296 A23 L297 L298 L299 L300 L301 L302 L303 L304 L305 L306 L307 L308 L309 L310 L311 L312 L313 L314 L316 L318 L319 L320 L323 A26 L325 L326 L327 L328 L329 L330 A27 L332 L333 L334 L335 L336 L353 L354 L355 L356 L357 L358 L359 L360 L361 L362 L363 L364 L365 L366 L367 L368 L369 L370 L371 L372 L373 L374 L375 L376 L377 L379 L380 L382 L383 L384 L546 L547 L548 L549 L550 L551 L552 L553 L554 L555 L556 L557 L558 L559 L562 L563 L565 A41 L566 A42 L573 L578 L581 L582 L585 L586 L587 L589 L590 L591 L592 L594 L596 L597 L598 L600 L601 L604 L605 L606 L608 L609 L610 L611 L612 L615 L644 L645 L647 L648 L649 L650 A48 L654 L655 L658 L659 L665 L666 L667 L668 L669 L670 L673 L675 L676 L677 L678 L679 L681 L682 L684 L686 A51 L687 L688 L690 L718 L720 L721 L725 L729 L735 L737 L747 L753 L765 L790 L881 L884 L939 L940 L941 L942 L943 L946 L950 L951 L953 A62 L960 L961 L964 L965 L968 L969 L970 L976 L978 L981 L987 A63 L988 L991 L992 L993 L997 L1000 L1002 L1003 L1006 L1007 L1009 L1011 L1012 L1014 L1036 L1056 L1060 L1068 L1276 L1314 L1322 L1346 A84 A86 L2359 A170 A183 L2892 L2893 L2894 L2895 L2896 L2897 L2898 L2899 L2900 L2901 L2902 L2903 L2904 L2905 L2906 A184 L2907 L2908 L2909 L2910 L2911 L2912 L2913 L2914 L2915 L2916 A185 L2917 L2918 L2919 L2920 L2921 L2922 L2923 L2924 L2925 L2926 L2927 L2928 L2929 L2930 L2931 L2932 L2933 L2934 L2935 L2936 L2937 L2938 L2939 L2940 L2941 L2942 L2943 A186 L2944 L2945 L2946 L2947 L2948 L2949 L2950 L2951 L2952 L2953 A187 L2954 L2955 L2956 L2957 L2958 L2959 L2960 L2961 L2962 L2963 L2964 L2965 L2966 L2967 L2968 L2969 L2970 L2971 L2972 L2973 L2974 L2975 L2976 L2977 L2978 L2979 L2980 A188 L2981 L2982 L2983 L2984 L2985 L2986 L2987 L2988 L2989 L2990 A189 L2991 L2992 L2993 L2994 L2995 L2996 L2997 L2998 L2999 L3000 L3001 L3002 L3003 L3004 L3005 A190 A225 | A8 A9 A10 A11 A190 A225 | L183 L184 L186 L189 L524 L529 L533 L534 L536 L540 L622 L626 L627 L630 L1260 L1262 L1267 L1292 L1318 L1367 L1448 L1477 L1692 L1702 L1704 L1708 L2402 L2405 L2416 L2419 L2424 L2425 L2427 L2428 L2430 L2432 | L263 L264 L265 L267 L269 L293 L378 L381 L426 L427 L431 L436 L437 L438 L439 L440 L444 L448 L449 L458 L461 L465 L483 L484 L485 L486 L487 L488 L489 L490 L491 L492 L493 L494 L495 L496 | L570 L717 L783 L880 L882 L885 L886 L887 L888 L889 L894 L895 L896 L897 L903 L923 L924 L925 L926 L927 L928 L938 L947 L948 L949 L952 L980 L982 L984 L994 L998 L1008 L1023 L1025 L1104 L1106 | L617 L996 L1010 L1031 L1043 L1070 L1394 L1395 L1399 L1406 L1432 L1472 L1510 L1512 L1525 L1558 L1559 L1561 L1566 L1691 L1694 L1707 L1712 L1727 L1744 L1774 L1781 L1785 L1793 L1806 L1816 L1878 L1885 L1908 L1909 L1914 | L623 L634 L660 L680 L954 L957 L972 L989 L995 L999 L1026 L1033 L1040 L1042 L1072 L1090 L1100 L1117 L1462 L1476 L2061 L2065 L2079 L2093 L2094 L2102 L2108 L2150 L2154 L2158 L2170 L2177 L2183 L2204 L2231 L2232 | L640 L657 L699 L708 L710 L719 L723 L731 L736 L742 L743 L744 L752 L785 L878 L890 L904 L910 L912 L916 L922 L932 L935 L936 L1015 L1021 L1027 L1053 L1061 L1073 L1256 L1258 L1259 L1272 L1288 L1316 | L642 L653 L661 L664 L694 L697 L704 L712 L722 L734 L842 L856 L1180 L1194 L1202 L1205 L1238 L1250 L1263 L1274 L1279 L1281 L1284 L1286 L1287 L1290 L1293 L1310 L1356 L1358 L1516 L1538 L1543 L1560 L1693 L1732 | L1965 L1996 L1999 L2000 L2001 L2005 L2008 L2018 L2019 L2020 L2022 L2043 L2044 L2052 L2054 L2058 L2059 L2068 L2070 L2083 L2087 L2090 L2101 L2109 L2110 L2112 L2127 L2128 L2132 L2145 L2146 L2168 L2187 L2203 L2219 L2222
sketch "Sketch3" plane through (-3, 0, 0) normal (-1, 0, 0) x (0, -1, 0)
  line L0 (0, -3) -> (0, 20)
  line L1 (0, 20) -> (-220, 20)
  line L2 (-220, 20) -> (-220, -3)
  line L3 (-220, -3) -> (0, -3)
  line L4 (4.62, -143.3562) -> (4.62, -141.9997)
  line L5 (1.72, -146.7368) -> (1.72, -144.4997)
  line L6 (7.0807, -146.0997) -> (4.42, -143.439)
  line L7 (4.42, -143.439) -> (4.42, -141.7997)
  line L8 (-0.1441, -94.3827) -> (-0.172, -94.4275)
  line L9 (4.42, -143.439) -> (4.42, -141.7997)
  line L10 (-0.0798, -94.2989) -> (-0.1133, -94.3397)
  line L11 (-0.0338, -94.5988) -> (-0.0478, -94.636)
  arc A0 (6.6572, -141.7997) -> (6.7986, -141.4582) centre (6.6572, -141.5997) ccw
  arc A1 (6.6572, -141.7997) -> (6.7986, -141.4582) centre (6.6572, -141.5997) ccw
  line L12 (3.2765, -144.6997) -> (5.82, -147.2432)
  arc A2 (1.2372, -147.0197) -> (1.92, -146.7368) centre (1.52, -146.7368) ccw
  line L13 (7.1635, -145.8997) -> (4.62, -143.3562)
  arc A3 (1.72, -93.2625) -> (1.3786, -93.1211) centre (1.52, -93.2625) ccw
  line L14 (-0.1969, -94.4741) -> (-0.2187, -94.5222)
  arc A4 (6.6572, -141.9997) -> (6.94, -141.3168) centre (6.6572, -141.5997) ccw
  line L15 (3.3593, -144.4997) -> (6.02, -147.1603)
  line L16 (-0.0459, -94.2627) -> (-0.0798, -94.2989)
  line L17 (-0.0683, -94.7127) -> (-0.0748, -94.7519)
  line L18 (0.0978, -94.4019) -> (0.0706, -94.4308)
  line L19 (-0.2187, -94.5222) -> (-0.2373, -94.5717)
  line L20 (1.92, -144.6997) -> (3.2765, -144.6997)
  line L21 (4.42, -141.7997) -> (6.6572, -141.7997)
  line L22 (7.0807, -146.0997) -> (4.42, -143.439)
  line L23 (-0.0174, -94.5626) -> (-0.0338, -94.5988)
  line L24 (-0.0748, -94.7519) -> (-0.0787, -94.7914)
  arc A5 (1.92, -93.2625) -> (1.2372, -92.9797) centre (1.52, -93.2625) ccw
  line L25 (3.3593, -144.4997) -> (6.02, -147.1603)
  line L26 (0.0454, -94.4616) -> (0.0223, -94.4938)
  line L27 (-0.0683, -94.7127) -> (-0.0748, -94.7519)
  line L28 (1.72, -146.7368) -> (1.72, -144.4997)
  line L29 (1.72, -144.4997) -> (3.3593, -144.4997)
  line L30 (4.62, -141.9997) -> (6.6572, -141.9997)
  line L31 (0.0454, -94.4616) -> (0.0223, -94.4938)
  arc A6 (1.72, -93.2625) -> (1.3786, -93.1211) centre (1.52, -93.2625) ccw
  line L32 (1.72, -144.4997) -> (3.3593, -144.4997)
  line L33 (0.0013, -94.5276) -> (-0.0174, -94.5626)
  line L34 (-0.0593, -94.674) -> (-0.0683, -94.7127)
  arc A7 (1.3786, -146.8782) -> (1.72, -146.7368) centre (1.52, -146.7368) ccw
  line L35 (4.42, -141.7997) -> (6.6572, -141.7997)
  line L36 (1.92, -146.7368) -> (1.92, -144.6997)
  arc A8 (1.3786, -146.8782) -> (1.72, -146.7368) centre (1.52, -146.7368) ccw
  line L37 (-0.2373, -94.5717) -> (-0.2526, -94.6222)
  line L38 (-0.0174, -94.5626) -> (-0.0338, -94.5988)
  line L39 (-0.0338, -94.5988) -> (-0.0478, -94.636)
  line L40 (-0.2646, -94.6736) -> (-0.2732, -94.7258)
  line L41 (-0.2526, -94.6222) -> (-0.2646, -94.6736)
  line L42 (1.3786, -93.1211) -> (0.0978, -94.4019)
  line L43 (1.2372, -92.9797) -> (-0.0459, -94.2627)
  line L44 (5.3921, -140.081) -> (5.357, -140.0623)
  line L45 (0.0978, -94.4019) -> (0.0706, -94.4308)
  line L46 (-0.1133, -94.3397) -> (-0.1441, -94.3827)
  line L47 (-0.0478, -94.636) -> (-0.0593, -94.674)
  line L48 (0.0706, -94.4308) -> (0.0454, -94.4616)
  line L49 (-0.172, -94.4275) -> (-0.1969, -94.4741)
  line L50 (0.0223, -94.4938) -> (0.0013, -94.5276)
  line L51 (-0.2732, -94.7258) -> (-0.2786, -94.7804)
  line L52 (0.0223, -94.4938) -> (0.0013, -94.5276)
  line L53 (0.0013, -94.5276) -> (-0.0174, -94.5626)
  line L54 (5.6207, -139.9999) -> (5.5799, -139.9663)
  line L55 (-0.0593, -94.674) -> (-0.0683, -94.7127)
  line L56 (-0.0787, -94.7914) -> (-0.08, -94.8997)
  line L57 (1.92, -95.2997) -> (1.92, -93.2625)
  line L58 (5.5799, -139.9663) -> (5.537, -139.9356)
  line L59 (5.537, -139.9356) -> (5.4921, -139.9077)
  line L60 (5.357, -139.9371) -> (5.3921, -139.9183)
  line L61 (1.3786, -93.1211) -> (0.0978, -94.4019)
  line L62 (-0.0787, -94.7914) -> (-0.08, -94.8997)
  line L63 (0.0706, -94.4308) -> (0.0454, -94.4616)
  line L64 (5.5178, -140.1775) -> (5.4888, -140.1503)
  line L65 (5.4581, -140.1251) -> (5.4258, -140.102)
  line L66 (5.3921, -140.081) -> (5.357, -140.0623)
  line L67 (1.72, -95.4997) -> (1.72, -93.2625)
  line L68 (5.4455, -140.1165) -> (5.4921, -140.0916)
  line L69 (5.4921, -139.9077) -> (5.4455, -139.8828)
  line L70 (-0.0478, -94.636) -> (-0.0593, -94.674)
  line L71 (6.02, -92.839) -> (3.3593, -95.4997)
  line L72 (5.2837, -139.9674) -> (5.3209, -139.9534)
  line L73 (5.357, -139.9371) -> (5.3921, -139.9183)
  line L74 (-0.0748, -94.7519) -> (-0.0787, -94.7914)
  line L75 (6.02, -92.839) -> (3.3593, -95.4997)
  line L76 (1.72, -95.4997) -> (1.72, -93.2625)
  line L77 (-0.2786, -94.7804) -> (-0.28, -94.8985)
  line L78 (5.4258, -139.8974) -> (5.4581, -139.8742)
  line L79 (5.3921, -139.9183) -> (5.4258, -139.8974)
  line L80 (5.82, -92.7562) -> (3.2765, -95.2997)
  line L81 (5.357, -140.0623) -> (5.3209, -140.0459)
  line L82 (5.3209, -139.9534) -> (5.357, -139.9371)
  line L83 (3.6807, -97.2997) -> (7.0807, -93.8997)
  line L84 (3.7635, -97.4997) -> (7.1635, -94.0997)
  line L85 (5.4888, -140.1503) -> (5.4581, -140.1251)
  line L86 (5.5799, -140.033) -> (5.6207, -139.9995)
  line L87 (-0.08, -94.8997) -> (-0.08, -105.0997)
  line L88 (-0.28, -94.8985) -> (-0.28, -105.1009)
  line L89 (3.6807, -97.2997) -> (7.0807, -93.8997)
  line L90 (5.4888, -140.1503) -> (5.4581, -140.1251)
  line L91 (5.4258, -139.8974) -> (5.4581, -139.8742)
  line L92 (5.4258, -140.102) -> (5.3921, -140.081)
  line L93 (7.0807, -106.0997) -> (3.6807, -102.6997)
  line L94 (7.1635, -105.8997) -> (3.7635, -102.4997)
  line L95 (5.4258, -140.102) -> (5.3921, -140.081)
  line L96 (7.0807, -106.0997) -> (3.6807, -102.6997)
  line L97 (5.2975, -140.1723) -> (5.348, -140.1569)
  line L98 (-0.08, -94.8997) -> (-0.08, -105.0997)
  line L99 (5.3921, -139.9183) -> (5.4258, -139.8974)
  line L100 (5.3974, -140.1383) -> (5.4455, -140.1165)
  line L101 (5.357, -140.0623) -> (5.3209, -140.0459)
  line L102 (5.5178, -140.1775) -> (5.4888, -140.1503)
  line L103 (5.1678, -140.0049) -> (5.1283, -140.001)
  line L104 (5.207, -139.988) -> (5.2457, -139.979)
  line L105 (5.3209, -140.0459) -> (5.2837, -140.0319)
  line L106 (5.4581, -140.1251) -> (5.4258, -140.102)
  line L107 (20.012, -85.5718) -> (20.0369, -85.5252)
  line L108 (19.8993, -85.3253) -> (19.9083, -85.2866)
  line L109 (5.537, -140.0637) -> (5.5799, -140.033)
  line L110 (5.3209, -140.0459) -> (5.2837, -140.0319)
  line L111 (20.0369, -85.5252) -> (20.0587, -85.4771)
  line L112 (5.6207, -139.9995) -> (5.6569, -139.9656)
  line L113 (20.0926, -85.3771) -> (20.1046, -85.3257)
  line L114 (5.4921, -140.0916) -> (5.537, -140.0637)
  line L115 (5.6569, -140.0337) -> (5.6207, -139.9999)
  line L116 (5.3209, -139.9534) -> (5.357, -139.9371)
  line L117 (5.2837, -139.9674) -> (5.3209, -139.9534)
  line L118 (5.348, -140.1569) -> (5.3974, -140.1383)
  line L119 (19.8574, -85.4367) -> (19.8738, -85.4005)
  line L120 (20.1046, -85.3257) -> (20.1132, -85.2736)
  line L121 (19.9841, -85.6166) -> (20.012, -85.5718)
  line L122 (19.8738, -85.4005) -> (19.8878, -85.3633)
  line L123 (19.7694, -85.5685) -> (19.7946, -85.5378)
  line L124 (19.8574, -85.4367) -> (19.8738, -85.4005)
  line L125 (20.0773, -85.4277) -> (20.0926, -85.3771)
  line L126 (5.2457, -139.979) -> (5.2837, -139.9674)
  line L127 (5.1283, -139.9984) -> (5.1678, -139.9945)
  line L128 (5.1413, -140.198) -> (5.1939, -140.1929)
  line L129 (19.7946, -85.5378) -> (19.8177, -85.5055)
  line L130 (5.1678, -139.9945) -> (5.207, -139.988)
  line L131 (5.1678, -140.0049) -> (5.1283, -140.001)
  line L132 (5.1939, -140.1929) -> (5.246, -140.1843)
  line L133 (5.1678, -139.9945) -> (5.207, -139.988)
  line L134 (19.8387, -85.4717) -> (19.8574, -85.4367)
  line L135 (5.207, -140.0113) -> (5.1678, -140.0049)
  line L136 (5.2457, -140.0203) -> (5.207, -140.0113)
  line L137 (20.1132, -85.2736) -> (20.1184, -85.221)
  line L138 (5.1283, -139.9984) -> (5.1678, -139.9945)
  line L139 (19.8878, -85.3633) -> (19.8993, -85.3253)
  line L140 (5.207, -139.988) -> (5.2457, -139.979)
  line L141 (19.9533, -85.6596) -> (19.9841, -85.6166)
  line L142 (19.8387, -85.4717) -> (19.8574, -85.4367)
  line L143 (5.2457, -140.0203) -> (5.207, -140.0113)
  line L144 (19.9083, -85.2866) -> (19.9148, -85.2474)
  line L145 (5.207, -140.0113) -> (5.1678, -140.0049)
  line L146 (19.8993, -85.3253) -> (19.9083, -85.2866)
  line L147 (19.8878, -85.3633) -> (19.8993, -85.3253)
  line L148 (5.2457, -139.979) -> (5.2837, -139.9674)
  line L149 (5.2837, -140.0319) -> (5.2457, -140.0203)
  line L150 (19.92, -154.8997) -> (19.9187, -154.7914)
  line L151 (19.9148, -154.7519) -> (19.9083, -154.7127)
  line L152 (16.1593, -157.2997) -> (18.12, -157.2997)
  line L153 (19.9187, -154.7914) -> (19.9148, -154.7519)
  line L154 (16.0765, -157.4997) -> (17.92, -157.4997)
  line L155 (13.82, -109.7998) -> (13.82, -107.1603)
  line L156 (20, -220) -> (20, 0)
  line L157 (6.02, -107.1603) -> (6.02, -109.7998)
  line L158 (6.02, -107.1603) -> (6.02, -109.7998)
  line L159 (19.9198, -154.2989) -> (19.8859, -154.2627)
  line L160 (19.8738, -154.5988) -> (19.8574, -154.5626)
  line L161 (19.9841, -154.3827) -> (19.9533, -154.3397)
  line L162 (19.8177, -154.4938) -> (19.7946, -154.4616)
  line L163 (19.9187, -154.7914) -> (19.9148, -154.7519)
  line L164 (13.82, -109.7998) -> (13.82, -107.1603)
  line L165 (20.1186, -154.7804) -> (20.1132, -154.7258)
  line L166 (19.8387, -154.5276) -> (19.8177, -154.4938)
  line L167 (19.8177, -154.4938) -> (19.7946, -154.4616)
  line L168 (-0.1969, -105.5252) -> (-0.172, -105.5718)
  arc A9 (19.42, -139.9997) -> (19.92, -139.4997) centre (19.42, -139.4997) ccw
  line L169 (14.5425, -139.8271) -> (14.492, -139.8424)
  line L170 (14.5191, -139.9534) -> (14.5563, -139.9674)
  line L171 (0.0706, -105.5685) -> (0.0978, -105.5975)
  line L172 (14.7482, -139.7997) -> (14.6987, -139.8013)
  line L173 (-0.0338, -105.4005) -> (-0.0174, -105.4367)
  arc A10 (19.42, -140.1997) -> (20.12, -139.4997) centre (19.42, -139.4997) ccw
  line L174 (0.0223, -105.5055) -> (0.0454, -105.5378)
  line L175 (14.4142, -139.8974) -> (14.4479, -139.9183)
  line L176 (-0.0174, -105.4367) -> (0.0013, -105.4717)
  line L177 (14.3819, -139.8742) -> (14.4142, -139.8974)
  line L178 (14.3819, -139.8742) -> (14.4142, -139.8974)
  line L179 (-0.1133, -105.6596) -> (-0.0798, -105.7004)
  line L180 (-0.0787, -105.2079) -> (-0.0748, -105.2474)
  line L181 (-0.2732, -105.2736) -> (-0.2646, -105.3257)
  line L182 (-0.0338, -105.4005) -> (-0.0174, -105.4367)
  line L183 (14.4142, -139.8974) -> (14.4479, -139.9183)
  line L184 (14.303, -139.9356) -> (14.2601, -139.9663)
  arc A11 (20.12, -140.4997) -> (19.42, -139.7997) centre (19.42, -140.4997) ccw
  line L185 (-0.0748, -105.2474) -> (-0.0683, -105.2866)
  arc A12 (19.42, -139.9997) -> (19.92, -139.4997) centre (19.42, -139.4997) ccw
  line L186 (14.5191, -139.9534) -> (14.5563, -139.9674)
  line L187 (14.4479, -139.9183) -> (14.483, -139.9371)
  line L188 (14.4426, -139.861) -> (14.3945, -139.8828)
  line L189 (14.492, -139.8424) -> (14.4426, -139.861)
  line L190 (3.3593, -104.4997) -> (6.02, -107.1603)
  line L191 (1.72, -106.7368) -> (1.72, -104.4997)
  arc A13 (1.2372, -107.0197) -> (1.92, -106.7368) centre (1.52, -106.7368) ccw
  line L192 (1.92, -106.7368) -> (1.92, -104.6997)
  line L193 (14.483, -139.9371) -> (14.5191, -139.9534)
  line L194 (14.3479, -139.9077) -> (14.303, -139.9356)
  line L195 (1.92, -104.6997) -> (3.2765, -104.6997)
  line L196 (14.3512, -139.849) -> (14.3819, -139.8742)
  line L197 (14.3222, -139.8219) -> (14.3512, -139.849)
  line L198 (14.4479, -139.9183) -> (14.483, -139.9371)
  line L199 (14.483, -139.9371) -> (14.5191, -139.9534)
  line L200 (3.2765, -104.6997) -> (5.82, -107.2432)
  line L201 (14.3512, -139.849) -> (14.3819, -139.8742)
  line L202 (1.72, -104.4997) -> (3.3593, -104.4997)
  line L203 (14.3222, -139.8219) -> (14.3512, -139.849)
  line L204 (3.3593, -104.4997) -> (6.02, -107.1603)
  line L205 (14.3945, -139.8828) -> (14.3479, -139.9077)
  line L206 (20.012, -154.4275) -> (19.9841, -154.3827)
  line L207 (19.9083, -154.7127) -> (19.8993, -154.674)
  line L208 (19.9533, -154.3397) -> (19.9198, -154.2989)
  line L209 (9.713, -86.0997) -> (7.0807, -86.0997)
  line L210 (18.12, -133.2625) -> (18.12, -135.4997)
  line L211 (13.82, -92.839) -> (13.82, -90.1995)
  line L212 (19.7694, -134.4308) -> (19.7422, -134.4019)
  line L213 (13.82, -92.839) -> (13.82, -90.1995)
  line L214 (6.02, -90.1995) -> (6.02, -92.839)
  line L215 (19.7422, -134.4019) -> (18.4614, -133.1211)
  circle A14 centre (9.92, -89.9997) radius 2.1
  arc A15 (18.4614, -133.1211) -> (18.12, -133.2625) centre (18.32, -133.2625) ccw
  line L216 (18.12, -135.4997) -> (16.4807, -135.4997)
  line L217 (18.12, -133.2625) -> (18.12, -135.4997)
  line L218 (19.7422, -134.4019) -> (18.4614, -133.1211)
  line L219 (17.92, -133.2625) -> (17.92, -135.2997)
  line L220 (9.713, -86.0997) -> (7.0807, -86.0997)
  line L221 (6.02, -90.1995) -> (6.02, -92.839)
  line L222 (18.12, -135.4997) -> (16.4807, -135.4997)
  line L223 (17.92, -135.2997) -> (16.5635, -135.2997)
  line L224 (5.82, -90.1167) -> (5.82, -92.7562)
  line L225 (14.02, -92.7562) -> (14.02, -90.1167)
  arc A16 (18.4614, -133.1211) -> (18.12, -133.2625) centre (18.32, -133.2625) ccw
  line L226 (-0.2526, -85.3771) -> (-0.2373, -85.4277)
  line L227 (0.0013, -85.4717) -> (0.0223, -85.5055)
  arc A17 (6.94, -138.6825) -> (6.6572, -137.9997) centre (6.6572, -138.3997) ccw
  line L228 (-0.08, -138.4997) -> (-0.08, -139.4997)
  line L229 (-0.08, -138.4997) -> (-0.08, -139.4997)
  line L230 (1.42, -139.7997) -> (0.42, -139.7997)
  line L231 (-0.1441, -85.6166) -> (-0.1133, -85.6596)
  line L232 (-0.28, -138.4997) -> (-0.28, -139.4997)
  arc A18 (-0.08, -139.4997) -> (0.42, -139.9997) centre (0.42, -139.4997) ccw
  line L233 (6.2199, -89.9997) -> (6.02, -90.1995)
  line L234 (5.5178, -139.8219) -> (6.7986, -138.5411)
  line L235 (5.0918, -139.7997) -> (1.42, -139.7997)
  line L236 (5.5178, -139.8219) -> (6.7986, -138.5411)
  arc A19 (6.7986, -138.5411) -> (6.6572, -138.1997) centre (6.6572, -138.3997) ccw
  line L237 (-0.2373, -85.4277) -> (-0.2187, -85.4771)
  line L238 (5.4455, -139.8828) -> (5.3974, -139.861)
  line L239 (5.4581, -139.8742) -> (5.4888, -139.849)
  line L240 (-0.0798, -85.7004) -> (-0.0459, -85.7366)
  line L241 (-0.2646, -85.3257) -> (-0.2526, -85.3771)
  line L242 (9.7981, -145.8997) -> (7.1635, -145.8997)
  line L243 (6.02, -147.1603) -> (6.02, -149.7998)
  line L244 (5.82, -147.2432) -> (5.82, -149.8826)
  line L245 (-0.0478, -85.3633) -> (-0.0338, -85.4005)
  line L246 (6.02, -147.1603) -> (6.02, -149.7998)
  line L247 (-0.0593, -85.3253) -> (-0.0478, -85.3633)
  arc A20 (-0.08, -139.4997) -> (0.42, -139.9997) centre (0.42, -139.4997) ccw
  line L248 (-0.1969, -85.5252) -> (-0.172, -85.5718)
  line L249 (5.4581, -139.8742) -> (5.4888, -139.849)
  line L250 (-0.0338, -85.4005) -> (-0.0174, -85.4367)
  line L251 (-0.2187, -85.4771) -> (-0.1969, -85.5252)
  line L252 (0.0978, -85.5975) -> (1.3786, -86.8782)
  line L253 (0.0454, -85.5378) -> (0.0706, -85.5685)
  line L254 (9.7152, -146.0997) -> (7.0807, -146.0997)
  arc A21 (0.42, -139.7997) -> (-0.28, -140.4997) centre (0.42, -140.4997) ccw
  line L255 (-0.1133, -85.6596) -> (-0.0798, -85.7004)
  line L256 (0.0013, -85.4717) -> (0.0223, -85.5055)
  line L257 (0.0706, -85.5685) -> (0.0978, -85.5975)
  line L258 (9.7152, -146.0997) -> (7.0807, -146.0997)
  arc A22 (-0.28, -139.4997) -> (0.42, -140.1997) centre (0.42, -139.4997) ccw
  line L259 (13.82, -149.7998) -> (13.82, -147.1603)
  arc A23 (1.2372, -87.0197) -> (1.92, -86.7368) centre (1.52, -86.7368) ccw
  line L260 (13.82, -149.7998) -> (13.82, -147.1603)
  line L261 (5.6569, -139.9656) -> (6.94, -138.6825)
  line L262 (-0.0174, -85.4367) -> (0.0013, -85.4717)
  line L263 (-0.0478, -85.3633) -> (-0.0338, -85.4005)
  line L264 (14.02, -149.8826) -> (14.02, -147.2432)
  line L265 (-0.0174, -85.4367) -> (0.0013, -85.4717)
  line L266 (0.0223, -85.5055) -> (0.0454, -85.5378)
  line L267 (0.0223, -85.5055) -> (0.0454, -85.5378)
  line L268 (0.0706, -85.5685) -> (0.0978, -85.5975)
  arc A24 (1.3786, -86.8782) -> (1.72, -86.7368) centre (1.52, -86.7368) ccw
  line L269 (0.0978, -85.5975) -> (1.3786, -86.8782)
  line L270 (-0.0593, -85.3253) -> (-0.0478, -85.3633)
  line L271 (0.0454, -85.5378) -> (0.0706, -85.5685)
  line L272 (-0.172, -85.5718) -> (-0.1441, -85.6166)
  arc A25 (1.3786, -86.8782) -> (1.72, -86.7368) centre (1.52, -86.7368) ccw
  line L273 (-0.0459, -85.7366) -> (1.2372, -87.0197)
  line L274 (-0.0338, -85.4005) -> (-0.0174, -85.4367)
  line L275 (19.8738, -134.5988) -> (19.8574, -134.5626)
  line L276 (4.62, -83.3562) -> (4.62, -81.9997)